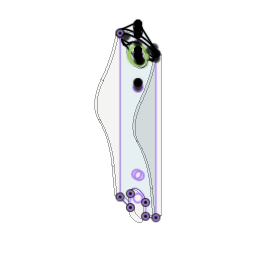
model (Autodesk Fusion 360 design; units mm, degrees)
Autodesk Fusion 360 part; units mm, degrees
sketch "side" plane through (0, 0, 0) normal (1, 0, 0) x (0, 1, 0) in component "plane"
  line L0 (0, 235) -> (0, 0)
  line L1 (0, 0) -> (-4.8, 0)
  line L2 (0, 235) -> (-4.8, 235)
  arc A0 (-4.8, 235) -> (-7.7294, 232.6468) centre (-4.8, 232) ccw
  arc A1 (-30.3403, 184.6468) -> (-7.7294, 232.6468) centre (-124.9072, 258.5189) ccw
  arc A2 (-30.3403, 184.6468) -> (-35.0106, 134.6468) centre (6.327, 156.0037) ccw
  arc A3 (-13.6574, 62.4184) -> (-35.0106, 134.6468) centre (-212.6974, 42.8458) ccw
  arc A4 (-7.7856, 2.7064) -> (-4.8, 0) centre (-4.8, 3) ccw
  line L3 (-7.7856, 2.7064) -> (-13.6574, 62.4184)
  line L4 (-40, 160.331) -> (0, 160.331) construction
  line L5 (-4.8, 235) -> (-4.8, 0)
  point P0 (-40, 160.331)
  dimension "d102" = 4.8
  dimension "d103" = 40
  dimension "d104" = 50
  dimension "d105" = 48
  dimension "d106" = 235
  dimension "d108" = 60
  dimension "d190" = 120
  dimension "d192" = 3
  dimension "d193" = 200
  constraint coincident L0.end L1.start
  constraint perpendicular L0 L1
  constraint perpendicular L0 L2
  constraint tangent L2 A0
  constraint tangent A0 A1
  constraint tangent A1 A2
  constraint tangent A2 A3
  constraint tangent L1 A4
  constraint tangent A3 L3
  constraint tangent A4 L3
  constraint vertical L0
  constraint equal A0 A4
  constraint equal L1 L2
  constraint midpoint A2 P0
  constraint coincident P0 L4.start
  constraint coincident L0 L4.end
  constraint perpendicular L0 L4
  measures "d102" distance of L0.start L2.end
  measures "d103" distance of P0 L4.end
  measures "d104" vertical distance of A1.start A2.end
  measures "d105" vertical distance of A0.end A1.start
  measures "d106" distance of L0.start L0.end
  measures "d108" distance of A3.start A4.start
  measures "d190" radius of A1
  measures "d192" radius of A0
  measures "d193" radius of A3
extrude "Extrude5" add sketch "side" along normal blind 62 in component "plane"
extrude "Extrude6" cut sketch "side" along normal blind 54.8 from surface at 3.6 contours A0 A1 A2 A3 A4 L3 L5 in component "plane"
sketch "bottom" plane through (0, 0, 0) normal (0, 1, 0) x (-1, 0, 0) in component "plane"
  line L0 (0, 0) -> (0, 235)
  line L1 (0, 235) -> (-62, 235)
  line L2 (-62, 235) -> (-62, 0)
  line L3 (-62, 0) -> (0, 0)
  arc A0 (0, 233) -> (-62, 233) centre (-31, 176.9375) ccw
  line L4 (-62, 233) -> (0, 233) construction
  arc A1 (-42.6, 11.6) -> (-19.4, 11.6) centre (-31, 11.6) ccw
  line L5 (-62, 20) -> (0, 20) construction
  circle A2 centre (-31, 219.5) radius 14.5
  line L6 (-31, 234) -> (-31, 241) construction
  line L7 (-31, 219.5) -> (-31, 234) construction
  arc A3 (-19.4, 30) -> (-42.6, 30) centre (-31, 30) ccw
  line L8 (-62, 20) -> (-92.9446, 31.2629) construction
  line L9 (0, 20) -> (39.2282, 34.2779) construction
  arc A4 (-19.4, 11.6) -> (0, 20) centre (-29.1181, 60.6465) ccw
  arc A5 (-62, 20) -> (-42.6, 11.6) centre (-32.8819, 60.6465) ccw
  line L10 (-19.4, 11.6) -> (-19.4, 30)
  line L11 (-42.6, 30) -> (-42.6, 11.6)
  line L12 (-31, 11.6) -> (-31, 30) construction
  line L13 (-19.4, 11.6) -> (0, 20) construction
  line L14 (-42.6, 11.6) -> (-62, 20) construction
  line L15 (-19.4, 11.6) -> (-31, 11.6) construction
  point P0 (-31, 241)
  point P1 (-31, 0)
  point P2 (-31, 234)
  point P3 (0, 235)
  dimension "d114" = 8
  dimension "d116" = 20
  dimension "d118" = 29
  dimension "d119" = 7
  dimension "d120" = 2
  dimension "d128" = 10
  dimension "d142" = 70
  dimension "d143" = 70
  dimension "d194" = 23.2
  dimension "d195" = 11.6
  dimension "d196" = 50
  constraint coincident L0 A0.start
  constraint coincident L2 A0.end
  constraint horizontal L4
  constraint midpoint A0 P0
  constraint coincident L2 L5.start
  constraint coincident L0 L5.end
  constraint horizontal L5
  constraint midpoint A1 P1
  constraint coincident L3 P1
  constraint coincident A2 P2
  constraint coincident P2 L6.start
  constraint coincident P0 L6.end
  constraint perpendicular L4 L6
  constraint coincident A2.centre L7.start
  constraint collinear L6 L7
  constraint equal A4 A5
  constraint vertical L10
  constraint coincident A1.centre L12.start
  constraint coincident A3.centre L12.end
  constraint vertical L12
  constraint equal L13 L14
  constraint equal A1 A3
  constraint horizontal L15
  measures "d114" distance of L4 P0
  measures "d116" vertical distance of L5.start P1
  measures "d118" diameter of A2
  measures "d119" distance of P2 P0
  measures "d120" distance of A0.start P3
  measures "d128" vertical distance of L5.end A3.start
  measures "d142" angle of L2 L8
  measures "d143" angle of L0 L9
  measures "d194" distance of L10 L11
  measures "d195" radius of A1
  measures "d196" radius of A5
extrude "Extrude7" add sketch "bottom" against normal up to surface (4.8 mm away) contours L1 A0 in component "plane"
extrude "Extrude8" cut sketch "bottom" against normal blind 80 contours L0 L3 A1 A4 | L2 L3 A1 A5 | L0 L1 A0 | L1 L2 A0 in component "plane"
extrude "Extrude9" add sketch "bottom" against normal blind 3 from surface at -4.8 contours A2 in component "plane"
extrude "Extrude10" add sketch "bottom" against normal up to surface (3 mm away) from surface at -4.8 contours A1 A3 L10 L11 in component "plane"
sketch "Sketch1" plane through (0, -4.8, 0) normal (0, -1, 0) x (1, 0, 0)
  circle A0 centre (31.001, 254) radius 7 construction
  circle A1 centre (31.001, 254) radius 2.25
  line L0 (3.6, 234.8447) -> (3.6, 240.8447) construction
  arc A2 (9.5815, 243.3134) -> (3.6, 234.8447) centre (12.5858, 234.8447) ccw
  line L1 (6.5915, 241.539) -> (26.3314, 259.2149)
  line L2 (31.001, 254) -> (31.001, 261) construction
  arc A3 (31.001, 261) -> (26.3314, 259.2149) centre (31.001, 254) ccw
  line L3 (31, 241) -> (31, 234) construction
  line L4 (58.4, 234.8447) -> (58.4, 240.8447) construction
  arc A4 (58.4, 240.8447) -> (3.6, 240.8447) centre (31, 182.9375) ccw construction
  line L5 (3.6, 234.8447) -> (3.6, 228.3388)
  line L6 (3.6, 228.3388) -> (9.2569, 222.682)
  line L7 (17.9185, 228.3388) -> (20.0398, 230.4602)
  arc A5 (31, 235) -> (20.0398, 230.4602) centre (31, 219.5) ccw
  circle A6 centre (31, 219.5) radius 14.5
  line L8 (17.9185, 228.3388) -> (3.6, 228.3388)
  line L9 (9.2569, 222.682) -> (12.2617, 222.682)
  line L10 (12.2617, 222.682) -> (17.9185, 228.3388)
  arc A7 (31, 247) -> (9.5815, 243.3134) centre (30.9725, 183.0972) ccw
  line L11 (31, 234) -> (31, 219.5) construction
  circle A8 centre (31, 219.5) radius 7 construction
  circle A9 centre (31, 219.5) radius 2.25
  line L12 (3.6, 228.3388) -> (27.2957, 213.5605)
  line L13 (31, 219.5) -> (31, 212.5) construction
  arc A10 (27.2957, 213.5605) -> (31, 212.5) centre (31, 219.5) ccw
  line L14 (55.4085, 241.539) -> (35.6686, 259.2149)
  arc A11 (35.6686, 259.2149) -> (30.999, 261) centre (30.999, 254) ccw
  arc A12 (58.4, 234.8447) -> (52.4185, 243.3134) centre (49.4142, 234.8447) ccw
  line L15 (58.4, 234.8447) -> (58.4, 228.3388)
  line L16 (44.0815, 228.3388) -> (58.4, 228.3388)
  line L17 (58.4, 228.3388) -> (52.7431, 222.682)
  line L18 (58.4, 228.3388) -> (34.7043, 213.5605)
  line L19 (52.7431, 222.682) -> (49.7383, 222.682)
  line L20 (49.7383, 222.682) -> (44.0815, 228.3388)
  arc A13 (41.9602, 230.4602) -> (31, 235) centre (31, 219.5) ccw
  line L21 (44.0815, 228.3388) -> (41.9602, 230.4602)
  arc A14 (52.4185, 243.3134) -> (31, 247) centre (31.0275, 183.0972) ccw
  arc A15 (58.4, 234.8447) -> (3.6, 234.8447) centre (31, 176.9375) ccw
  line L22 (19.4, 11.6) -> (19.4, 30)
  arc A16 (42.6, 30) -> (19.4, 30) centre (31, 30) ccw
  line L23 (42.6, 30) -> (42.6, 11.6)
  arc A17 (42.6, 11.6) -> (58.4, 17.6485) centre (32.8819, 60.6465) ccw
  line L24 (58.4, 17.6485) -> (58.4, 234.8447)
  arc A18 (58.4, 234.8447) -> (3.6, 234.8447) centre (31, 176.9375) ccw
  line L25 (3.6, 234.8447) -> (3.6, 17.6485)
  arc A19 (3.6, 17.6485) -> (19.4, 11.6) centre (29.1181, 60.6465) ccw
  circle A20 centre (31, 219.5) radius 14.5
  arc A21 (31, 212.5) -> (34.7043, 213.5605) centre (31, 219.5) ccw
  point P0 (31, 247)
  point P1 (3.6, 234.8447)
  point P2 (31.001, 261)
  point P3 (31, 219.5)
  point P4 (31, 226.5)
  dimension "d197" = 14
  dimension "d198" = 4.5
  dimension "d199" = 6
  dimension "d201" = 8
  dimension "d202" = 1
  dimension "d203" = 3
  dimension "d204" = 45
  dimension "d205" = 135
  dimension "d206" = 6.5059
  dimension "d207" = 7.5
  constraint coincident A0 P0
  constraint concentric A0 A1
  constraint vertical L0
  constraint coincident L0 P1
  constraint tangent L0 A2
  constraint coincident A0 L1.end
  constraint tangent A0 L1
  constraint coincident A0 P2
  constraint coincident A0.centre A1.centre
  constraint coincident P2 L2.end
  constraint vertical L2
  constraint tangent L1 A3
  constraint vertical L3
  constraint symmetric P1 L3 L4.start
  constraint symmetric L0.end L3 L4.end
  constraint tangent A2 A4
  constraint coincident A4 A2.start
  constraint tangent A2 L1
  constraint coincident L1.start A2
  constraint midpoint P0 A4
  constraint tangent A0 A4
  constraint coincident P1 L0.start
  constraint tangent A2 L5
  constraint coincident L3 A5.start
  constraint coincident P3 A5.centre
  constraint coincident L3.end A6
  constraint coincident L5 L6.start
  constraint coincident L5.end L6.start
  constraint horizontal L8
  constraint horizontal L9
  constraint equal L6 L10
  constraint tangent A0 A7
  constraint coincident P0 A7.start
  constraint parallel L3 L11
  constraint concentric A8 A9
  constraint equal A0 A8
  constraint equal A1 A9
  constraint tangent L7 A5
  constraint coincident A8 P4
  constraint coincident L11 P4
  constraint coincident A8 L12.end
  constraint tangent A8 L12
  constraint coincident A8 L13.end
  constraint vertical L13
  constraint tangent L12 A10
  constraint symmetric L1.start L3 L14.start
  constraint symmetric A2 L3 A12
  constraint symmetric L1.end L3 L14.end
  constraint symmetric P2 L3 A11.end
  constraint symmetric A3 L3 A11
  constraint symmetric L3 A2.start A12.end
  constraint symmetric L3 P1 L4.start
  constraint symmetric L3 L5.end L15.end
  constraint symmetric L3 L6.end L17.end
  constraint symmetric L3 L7.start L16.start
  constraint symmetric L3 L7.end A13.start
  constraint symmetric L3 A5.start A13.end
  constraint symmetric L3 A5 A13
  constraint symmetric L3 L9.end L19.end
  constraint symmetric L3 P0 A7.start
  constraint symmetric L3 A7 A14
  constraint symmetric L3 L12.end L18.end
  constraint coincident L3.start A15
  constraint equal A15 A18
  constraint symmetric L3 L13.end A10.end
  constraint symmetric L3 A10 A21
  measures "d197" diameter of A0
  measures "d198" diameter of A1
  measures "d199" distance of L0.end P1
  measures "d201" distance of L5.end L6.end
  measures "d202" distance of L3.end A5.start
  measures "d203" distance of L7.start L7.end
  measures "d204" angle of L6 L8
  measures "d205" angle of L7 L8
  measures "d206" distance of P1 L5.end
  measures "d207" distance of L3.end P4
sketch "Sketch2" plane through (0, -4.8, 0) normal (0, -1, 0) x (1, 0, 0) in component "bot"
  line L0 (58.4, 17.6485) -> (58.4, 234.8447)
  arc A0 (58.4, 234.8447) -> (3.6, 234.8447) centre (31, 176.9375) ccw
  line L1 (3.6, 234.8447) -> (3.6, 17.6485)
  arc A1 (42.6, 30) -> (19.4, 30) centre (31, 30) ccw
  circle A2 centre (31, 219.5) radius 14.5
  line L2 (3.85, 48.5181) -> (3.85, 54.5181)
  line L3 (19.15, 33.9825) -> (19.15, 27.9825)
  arc A3 (19.15, 33.9825) -> (3.85, 54.5181) centre (-6.8452, 30.5823) ccw
  arc A4 (6.0901, 53.3855) -> (3.85, 52.0808) centre (5.35, 52.0808) ccw
  line L4 (3.6, 17.6485) -> (3.6, 62.4184)
  line L5 (3.85, 48.6682) -> (3.6, 48.6682) construction
  line L6 (19.15, 42.3966) -> (19.4, 42.3966) construction
  line L7 (3.85, 48.5181) -> (3.85, 40.5181)
  line L8 (19.15, 27.9825) -> (19.15, 19.9825)
  arc A5 (19.15, 19.9825) -> (3.85, 40.5181) centre (-6.8452, 16.5823) ccw
  line L9 (19.4, 30) -> (42.6, 30) construction
  line L10 (31, 30) -> (31, 41.6) construction
  line L11 (31, 30) -> (31, 0) construction
  line L12 (19.15, 19.9825) -> (31, 19.9825)
  line L13 (3.85, 48.5181) -> (31, 48.5181)
  circle A6 centre (25.2, 34.2503) radius 2.25
  circle A7 centre (25.2, 34.2503) radius 6.25 construction
  line L14 (31, 48.5181) -> (25.2, 34.2503) construction
  line L15 (25.2, 34.2503) -> (31, 19.9825) construction
  line L16 (25.2, 34.2503) -> (19.4, 48.5181) construction
  arc A8 (58.15, 54.5181) -> (42.85, 33.9825) centre (68.8452, 30.5823) ccw
  arc A9 (58.15, 52.0808) -> (55.9099, 53.3855) centre (56.65, 52.0808) ccw
  line L17 (58.15, 48.5181) -> (58.15, 54.5181)
  line L18 (58.15, 48.5181) -> (58.15, 40.5181)
  arc A10 (58.15, 40.5181) -> (42.85, 19.9825) centre (68.8452, 16.5823) ccw
  line L19 (42.85, 33.9825) -> (42.85, 27.9825)
  line L20 (42.85, 27.9825) -> (42.85, 19.9825)
  circle A11 centre (36.8, 34.2503) radius 2.25
  line L21 (58.15, 48.5181) -> (31, 48.5181)
  line L22 (42.85, 19.9825) -> (31, 19.9825)
  line L23 (18.8498, 19.9825) -> (19.4, 11.6)
  line L24 (42.6, 19.9825) -> (42.6, 11.6)
  line L25 (19.4, 11.6) -> (19.4, 30)
  line L26 (42.6, 30) -> (42.6, 11.6)
  arc A12 (42.6, 11.6) -> (58.4, 17.6485) centre (32.8819, 60.6465) ccw
  arc A13 (3.6, 17.6485) -> (19.4, 11.6) centre (29.1181, 60.6465) ccw
  dimension "d164" = 1.5
  dimension "d165" = 0.25
  dimension "d167" = 6
  dimension "d168" = 8
  dimension "d169" = 4.5
  dimension "d170" = 12.5
  constraint parallel L1 L2
  constraint parallel L2 L3
  constraint equal L2 L3
  constraint tangent L2 A4
  constraint coincident A3 A4.start
  constraint coincident L2 A4.end
  constraint tangent A3 A4
  constraint coincident L2 L5.start
  constraint coincident L1 L5.end
  constraint perpendicular L1 L5
  constraint coincident L3 L6.start
  constraint equal L5 L6
  constraint parallel L4 L7
  constraint equal L7 L8
  constraint equal A3 A5
  constraint coincident A1.end L9.start
  constraint coincident A1.start L9.end
  constraint coincident A1.centre L10.start
  constraint midpoint A1 L10.end
  constraint perpendicular L9 L11
  constraint coincident L11 L12.end
  constraint perpendicular L11 L12
  constraint coincident L11 L13.end
  constraint perpendicular L11 L13
  constraint concentric A6 A7
  constraint coincident A6.centre A7.centre
  constraint coincident L13 L16.end
  constraint equal L14 L16
  constraint equal L14 L15
  constraint symmetric L2.start L11 L17.start
  constraint symmetric L2.end L11 A8.start
  constraint symmetric L3.start L11 A8.end
  constraint symmetric L3.end L11 L19.end
  constraint symmetric A3 L11 A8
  constraint symmetric A4.end L11 A9.start
  constraint symmetric A4.start L11 A9.end
  constraint symmetric A4 L11 A9
  constraint symmetric L7.end L11 L18.end
  constraint symmetric L8.end L11 A10.end
  constraint symmetric A5 L11 A10
  constraint symmetric L11 L12.end L15.end
  constraint symmetric L11 L13.end L14.start
  constraint symmetric L11 A6 A11
  constraint coincident L12 L23.start
  constraint coincident L22 L24.start
  constraint vertical L24
  measures "d164" radius of A4
  measures "d165" distance of L2 L4
  measures "d167" distance of L2.start L2.end
  measures "d168" distance of L2.start L7.end
  measures "d169" diameter of A6
  measures "d170" diameter of A7
extrude "Extrude5'" [suppressed] in component "bot"
extrude "Extrude6'" [suppressed] in component "bot"
extrude "Extrude7'" [suppressed] in component "bot"
fillet "Fillet2" [suppressed] in component "bot"
chamfer "Chamfer6" [suppressed] in component "bot"
component "plane" placed x (1, 0, 0) y (0, 1, 0) z (0, 0, 1) at (0, 0, 0)
component "top" placed x (1, 0, 0) y (0, 1, 0) z (0, 0, 1) at (0, 0, 0)
component "bot" placed x (1, 0, 0) y (0, 1, 0) z (0, 0, 1) at (0, 0, 0)
equation "outerWidth = 62 mm"
equation "innerWidth = outerWidth - 7.2 mm"
equation "baseThickness = 4.8 mm"
equation "arcDepth = 8 mm"
equation "totalLength = 235 mm"
equation "frontHumpOffset = 48 mm"
equation "humpLength = 50 mm"
equation "humpHeight = 40 mm"
equation "knobFrontInset = 7 mm"
equation "mountThickness = 8 mm"
equation "screwOD = 10 mm"
equation "screwID = 4.5 mm"
equation "screwChamfer = 4 mm"
equation "toteExtension = 20 mm"
equation "toteExtensionWidth = 23.2 mm"
equation "d102 = baseThickness"
equation "d103 = humpHeight"
equation "d104 = humpLength"
equation "d105 = frontHumpOffset"
equation "d106 = totalLength"
equation "d109 = outerWidth"
equation "d111 = ( outerWidth - innerWidth ) / 2"
equation "d112 = innerWidth"
equation "d114 = arcDepth"
equation "d116 = toteExtension"
equation "knobDiameter = 29 mm"
equation "d118 = knobDiameter"
equation "d119 = knobFrontInset"
equation "d143 = d142"
equation "d194 = toteExtensionWidth"
equation "d195 = d194 / 2"
equation "d197 = screwOD + 4 mm"
equation "d198 = screwID"
